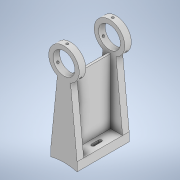
# Autodesk Inventor part: finderV03
Saved by Autodesk Inventor 2020.3 (Build 243373000, 373)
## iProperties
Created: 2020-06-05
Part Number: finderV03
Material: Generic
Document SubType Name: Modeling
Designer: robst
Density: 1 g/cm^3
Appearance: Default
Author: robst
Autodesk Inventor part; units mm, degrees
ref_plane "YZ Plane" through (0, 0, 0) normal (1, 0, 0) x (0, 1, 0)
ref_plane "XY Plane" through (0, 0, 0) normal (0, 0, 1) x (1, 0, 0)
sketch "Sketch1" plane through (0, 0, 0) normal (0, 0, 1) x (1, 0, 0)
  arc A0 (19.05, 73.7803) -> (-19.05, 73.7803) centre (0, 0) ccw
  line L0 (0, 86.4803) -> (19.05, 86.4803)
  line L1 (19.05, 86.4803) -> (19.05, 73.7803)
  line L2 (0, 76.2) -> (0, 86.4803) construction
  line L3 (0, 86.4803) -> (-19.05, 86.4803)
  line L4 (-19.05, 86.4803) -> (-19.05, 73.7803)
  dimension "d0" = 152.4
  dimension "d1" = 19.05
  dimension "d2" = 12.7
  constraints: 10 end point, 3 point on circle, 2 symmetric about line, 1 centre point, 1 coincident, 1 horizontal, 1 perpendicular, 1 vertical
  measures "d0" diameter of A0
  measures "d1" distance of L0.start L0.end
  measures "d2" distance of L0.end L1.end
extrude "Extrusion1" add sketch "Sketch1" along normal mid plane 75.6666
sketch "Sketch2" plane through (-19.05, 86.4803, 37.8333) normal (0, 1, 0) x (1, 0, 0)
  line L0 (0, 75.6666) -> (0, 0) construction
  line L1 (0, 37.8333) -> (38.1, 37.8333) construction
  line L2 (38.1, 75.6666) -> (38.1, 0) construction
  line L3 (0, 75.6666) -> (38.1, 75.6666) construction
  line L4 (19.05, 75.6666) -> (19.05, 0) construction
  line L5 (38.1, 0) -> (0, 0) construction
  line L6 (28.575, 32.4358) -> (28.575, 43.2308) construction
  line L7 (26.3525, 32.4358) -> (26.3525, 43.2308)
  line L8 (30.7975, 43.2308) -> (30.7975, 32.4358)
  arc A0 (26.3525, 32.4358) -> (30.7975, 32.4358) centre (28.575, 32.4358) ccw
  arc A1 (30.7975, 43.2308) -> (26.3525, 43.2308) centre (28.575, 43.2308) ccw
  line L9 (11.7475, 32.4358) -> (11.7475, 43.2308)
  line L10 (7.3025, 43.2308) -> (7.3025, 32.4358)
  arc A2 (7.3025, 32.4358) -> (11.7475, 32.4358) centre (9.525, 32.4358) ccw
  arc A3 (11.7475, 43.2308) -> (7.3025, 43.2308) centre (9.525, 43.2308) ccw
  point P0 (19.05, 37.8333)
  point P1 (28.575, 37.8333)
  dimension "d5" = 9.525
  dimension "d6" = 4.445
  dimension "d7" = 15.24
  dimension "d8" = 19.05
  constraints: 16 end point, 8 point on circle, 6 symmetric about line, 5 midpoint, 4 centre point, 4 tangent, 1 parallel, 1 perpendicular, 1 point on line, 2 other
  measures "d5" distance of point (28.575, 37.833) point (19.05, 37.833)
  measures "d6" distance between parallel lines of L8 L7
  measures "d8" distance of L6.end A3.centre
extrude "Extrusion2" cut sketch "Sketch2" against normal through all
ref_plane "Work Plane1" through (19.05, 73.7803, 37.8333) normal (0, 1, 0) x (-1, 0, 0)
sketch "Sketch4" plane through (19.05, 73.7803, 37.8333) normal (0, 1, 0) x (-1, 0, 0)
  line L0 (11.7475, -43.2308) -> (11.7475, -32.4358) projected
  line L1 (11.7475, -32.4358) -> (11.7475, -43.2308) construction
  line L2 (11.7475, -37.8333) -> (7.3025, -37.8333) construction
  line L3 (7.3025, -43.2308) -> (7.3025, -32.4358) construction
  line L4 (9.525, -42.2783) -> (9.525, -33.3883) construction
  line L5 (14.605, -42.2783) -> (14.605, -33.3883)
  line L6 (4.445, -33.3883) -> (4.445, -42.2783)
  arc A0 (4.445, -42.2783) -> (14.605, -42.2783) centre (9.525, -42.2783) ccw
  arc A1 (14.605, -33.3883) -> (4.445, -33.3883) centre (9.525, -33.3883) ccw
  line L7 (0, 0) -> (38.1, 0) construction
  line L8 (19.05, 0) -> (19.05, -75.6666) construction
  line L9 (38.1, -75.6666) -> (0, -75.6666) construction
  line L10 (23.495, -42.2783) -> (23.495, -33.3883)
  line L11 (33.655, -33.3883) -> (33.655, -42.2783)
  arc A2 (23.495, -42.2783) -> (33.655, -42.2783) centre (28.575, -42.2783) ccw
  arc A3 (33.655, -33.3883) -> (23.495, -33.3883) centre (28.575, -33.3883) ccw
  point P0 (19.05, -37.8333)
  point P1 (9.525, -37.8333)
  dimension "d11" = 10.16
  dimension "d12" = 19.05
  constraints: 16 end point, 8 point on circle, 6 midpoint, 6 symmetric about line, 4 centre point, 4 tangent, 1 parallel, 1 perpendicular, 2 other
  measures "d11" distance between parallel lines of L6 L5
extrude "Extrusion3" cut sketch "Sketch4" along normal blind 7.62
sketch "Sketch5" plane through (0, 0, 37.8333) normal (0, 0, 1) x (1, 0, 0)
  circle A0 centre (0, 200.7803) radius 15.875
  arc A1 (9.525, 180.6999) -> (-9.525, 180.6999) centre (0, 200.7803) ccw
  arc A2 (19.05, 73.7803) -> (-19.05, 73.7803) centre (0, 0) ccw construction
  line L0 (-19.05, 73.7803) -> (19.05, 73.7803) construction
  line L1 (19.05, 86.4803) -> (9.525, 180.6999)
  line L2 (19.05, 86.4803) -> (-19.05, 86.4803) construction
  line L3 (0, 86.4803) -> (0, 200.7803) construction
  line L4 (-19.05, 86.4803) -> (-9.525, 180.6999)
  line L5 (-19.05, 86.4803) -> (19.05, 86.4803)
  dimension "d15" = 31.75
  dimension "d16" = 6.35
  dimension "d17" = 127
  dimension "d18" = 9.525
  constraints: 10 end point, 2 centre point, 2 horizontal, 2 point on circle, 1 coincident, 1 midpoint, 1 perpendicular, 1 symmetric about line
  measures "d15" diameter of A0
  measures "d16" radial gap between concentric circles of A1 A0
  measures "d17" distance from line of A0.centre L0
  measures "d18" distance from line of L1.end L3
extrude "Extrusion4" add sketch "Sketch5" against normal blind 9.525
ref_plane "Work Plane2" through (0, 223.0053, 37.8333) normal (0, 1, 0) x (-1, 0, 0)
sketch "Sketch6" plane through (0, 223.0053, 37.8333) normal (0, 1, 0) x (-1, 0, 0)
  line L0 (-22.225, -9.525) -> (22.225, -9.525) projected
  circle A0 centre (0, -4.7625) radius 1.7272
  point P0 (0, -37.8333)
  point P1 (9.525, -9.525)
  point P2 (-9.525, -9.525)
  dimension "d21" = 4.7625
  dimension "d22" = 3.4544
  constraints: 1 centre point
  measures "d21" distance from line of A0.centre L0
  measures "d22" diameter of A0
extrude "Extrusion5" cut sketch "Sketch6" against normal up to surface round surface about axis through (0, 200.7803, 37.8333) along (0, 0, -1) radius 15.875 far side no
pattern_circular "Circular Pattern1" count 3 over 360 about axis through (0, 200.7803, 37.8333) along (0, 0, -1) of "Extrusion5"
mirror "Mirror1" about plane through (0, 0, 0) normal (0, 0, 1) of "Extrusion4", "Extrusion5", "Circular Pattern1"
sketch "Sketch7" plane through (0, 0, 0) normal (1, 0, 0) x (0, 1, 0)
  line L0 (86.4803, 28.3083) -> (180.6999, 28.3083) projected
  line L1 (180.6999, -28.3083) -> (86.4803, -28.3083) projected
  line L2 (86.4803, 28.3083) -> (180.6999, 28.3083)
  line L3 (180.6999, 28.3083) -> (180.6999, -28.3083)
  line L4 (180.6999, -28.3083) -> (86.4803, -28.3083)
  line L5 (86.4803, -28.3083) -> (86.4803, 28.3083)
  point P0 (0, 0)
  constraints: 8 end point, 2 parallel, 1 horizontal, 1 perpendicular
extrude "Extrusion6" add sketch "Sketch7" along normal mid plane 3.175
body "Solid1"
